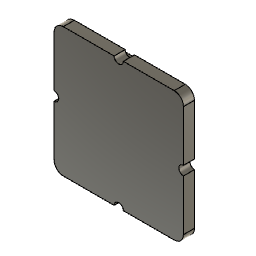
Coaster Holder with Coaster v3 (Autodesk Fusion 360 archive; units mm, degrees)
design "Coaster"
Autodesk Fusion 360 part; units mm, degrees
sketch "Sketch3" plane through (0, 0, 0) normal (0, 1, 0) x (1, 0, 0)
  line L0 (127, -127) -> (38.1, -127)
  line L1 (38.1, -127) -> (38.1, -38.1)
  line L2 (38.1, -38.1) -> (127, -38.1)
  line L3 (127, -38.1) -> (127, -127)
  line L4 (127, -82.55) -> (38.1, -82.55) construction
  dimension "d24" = 88.9
  dimension "d25" = 88.9
  constraint horizontal L0
  constraint vertical L1
  constraint horizontal L2
  constraint vertical L3
  constraint midpoint L3 L4.start
  constraint midpoint L1 L4.end
  measures "d24" distance of L0.start L0.end
  measures "d25" distance of L0.start L2.end
sketch "Sketch4" plane through (0, 0, 0) normal (0, 1, 0) x (1, 0, 0)
  line L0 (114.3445, -111.3227) -> (104.4288, -120.5494)
  line L1 (104.4288, -120.5494) -> (60.6138, -120.5494)
  line L2 (60.6138, -120.5494) -> (50.4318, -111.0618)
  line L3 (50.4318, -111.0618) -> (50.4318, -98.4259)
  line L4 (50.4318, -98.4259) -> (65.3763, -98.4259)
  line L5 (65.3763, -98.4259) -> (65.3763, -106.5936)
  line L6 (65.3763, -106.5936) -> (99.367, -106.5936)
  line L7 (99.367, -106.5936) -> (99.367, -90.3353)
  line L8 (99.367, -90.3353) -> (60.7032, -90.3353)
  line L9 (60.7032, -90.3353) -> (50.5442, -80.8012)
  line L10 (50.5442, -80.8012) -> (50.5442, -54.1925)
  line L11 (50.5442, -54.1925) -> (60.7032, -44.5506)
  line L12 (60.7032, -44.5506) -> (104.4543, -44.5506)
  line L13 (104.4543, -44.5506) -> (114.6143, -54.0756)
  line L14 (114.6143, -54.0756) -> (114.6143, -66.7756)
  line L15 (114.6143, -66.7756) -> (99.3743, -66.7756)
  line L16 (99.3743, -66.7756) -> (99.3108, -58.7746)
  line L17 (99.3108, -58.7746) -> (65.7193, -58.7746)
  line L18 (65.7193, -58.7746) -> (65.7193, -76.3006)
  line L19 (65.7193, -76.3006) -> (104.4543, -76.3006)
  line L20 (104.4543, -76.3006) -> (114.4555, -85.8256)
  line L21 (114.4555, -85.8256) -> (114.3445, -111.3227)
  line L22 (82.5213, -120.5494) -> (82.5787, -44.5506) construction
  line L23 (127, -82.55) -> (38.1, -82.55)
  constraint horizontal L12
  constraint midpoint L1 L22.start
  constraint midpoint L12 L22.end
  constraint midpoint L22 L23
extrude "Extrude5" add sketch "Sketch4" along normal blind 12.7 makes body 1
extrude "Extrude6" cut sketch "Sketch3" along normal blind 5.08 bodies 1
extrude "Extrude7" add sketch "Sketch4" sketch "Sketch3" along normal blind 7.62 of sketch 2 bodies 1
scale "Scale1" factor 1 about (127, 7.62, 127) bodies 1
sketch "Sketch7" plane through (0, 7.62, 0) normal (0, 1, 0) x (-1, 0, 0)
  line L0 (-127, 38.1) -> (-38.1, 38.1)
  line L1 (-38.1, 38.1) -> (-38.1, 127)
  line L2 (-38.1, 127) -> (-127, 127)
  line L3 (-127, 127) -> (-127, 38.1)
  line L4 (-50.5442, 80.8012) -> (-50.5442, 54.1925)
  line L5 (-50.5442, 54.1925) -> (-60.7032, 44.5506)
  line L6 (-60.7032, 44.5506) -> (-104.4543, 44.5506)
  line L7 (-104.4543, 44.5506) -> (-114.6143, 54.0756)
  line L8 (-114.6143, 54.0756) -> (-114.6143, 66.7756)
  line L9 (-114.6143, 66.7756) -> (-99.3743, 66.7756)
  line L10 (-99.3743, 66.7756) -> (-99.3108, 58.7746)
  line L11 (-99.3108, 58.7746) -> (-65.7193, 58.7746)
  line L12 (-65.7193, 58.7746) -> (-65.7193, 76.3006)
  line L13 (-65.7193, 76.3006) -> (-104.4543, 76.3006)
  line L14 (-104.4543, 76.3006) -> (-114.4555, 85.8256)
  line L15 (-114.4555, 85.8256) -> (-114.3445, 111.3227)
  line L16 (-114.3445, 111.3227) -> (-104.4288, 120.5494)
  line L17 (-104.4288, 120.5494) -> (-60.6138, 120.5494)
  line L18 (-60.6138, 120.5494) -> (-50.4318, 111.0618)
  line L19 (-50.4318, 111.0618) -> (-50.4318, 98.4259)
  line L20 (-50.4318, 98.4259) -> (-65.3763, 98.4259)
  line L21 (-65.3763, 98.4259) -> (-65.3763, 106.5936)
  line L22 (-65.3763, 106.5936) -> (-99.367, 106.5936)
  line L23 (-99.367, 106.5936) -> (-99.367, 90.3353)
  line L24 (-99.367, 90.3353) -> (-60.7032, 90.3353)
  line L25 (-60.7032, 90.3353) -> (-50.5442, 80.8012)
  line L26 (-127, 82.55) -> (-38.1, 82.55) construction
  line L27 (-82.55, 127) -> (-82.55, 38.1) construction
  circle A0 centre (-127, 82.55) radius 3.175
  circle A1 centre (-82.55, 127) radius 3.175
  circle A2 centre (-38.1, 82.55) radius 3.175
  circle A3 centre (-82.55, 38.1) radius 3.175
  dimension "d33" = 6.35
  dimension "d34" = 6.35
  dimension "d35" = 6.35
  dimension "d36" = 6.35
  constraint midpoint L3 L26.start
  constraint midpoint L1 L26.end
  constraint midpoint L2 L27.start
  constraint midpoint L0 L27.end
  constraint coincident L26.start A0.centre
  constraint coincident L27.start A1.centre
  constraint coincident L26.end A2.centre
  constraint coincident L27.end A3.centre
  measures "d33" diameter of A0
  measures "d34" diameter of A1
  measures "d35" diameter of A2
  measures "d36" diameter of A3
extrude "Extrude8" cut sketch "Sketch7" against normal blind 25.4 contours L0 A3 | L0 A3 | L1 A2 | L1 A2 | L3 A0 | L3 A0 | L2 A1 | L2 A1 bodies 1
fillet "Fillet2" radius 6.35 4 edges at (38.1, 3.81, 38.1) (38.1, 3.81, 127) (127, 3.81, 127) (127, 3.81, 38.1) on bodies 1
copy_body "Body->Comp1" bodies 1 removing the originals makes body 2 in component "Coaster"
sketch "Sketch8" plane through (0, 7.62, 0) normal (0, 1, 0) x (-1, 0, 0)
  arc A0 (-127, 44.45) -> (-120.65, 38.1) centre (-120.65, 44.45) ccw
  line L0 (-120.65, 38.1) -> (-85.725, 38.1)
  arc A1 (-79.375, 38.1) -> (-85.725, 38.1) centre (-82.55, 38.1) ccw
  line L1 (-79.375, 38.1) -> (-44.45, 38.1)
  arc A2 (-44.45, 38.1) -> (-38.1, 44.45) centre (-44.45, 44.45) ccw
  line L2 (-38.1, 44.45) -> (-38.1, 79.375)
  arc A3 (-38.1, 85.725) -> (-38.1, 79.375) centre (-38.1, 82.55) ccw
  line L3 (-38.1, 85.725) -> (-38.1, 120.65)
  arc A4 (-38.1, 120.65) -> (-44.45, 127) centre (-44.45, 120.65) ccw
  line L4 (-44.45, 127) -> (-79.375, 127)
  arc A5 (-85.725, 127) -> (-79.375, 127) centre (-82.55, 127) ccw
  line L5 (-85.725, 127) -> (-120.65, 127)
  arc A6 (-120.65, 127) -> (-127, 120.65) centre (-120.65, 120.65) ccw
  line L6 (-127, 120.65) -> (-127, 85.725)
  arc A7 (-127, 79.375) -> (-127, 85.725) centre (-127, 82.55) ccw
  line L7 (-127, 79.375) -> (-127, 44.45)
  line L8 (-50.5442, 80.8012) -> (-50.5442, 54.1925)
  line L9 (-50.5442, 54.1925) -> (-60.7032, 44.5506)
  line L10 (-60.7032, 44.5506) -> (-104.4543, 44.5506)
  line L11 (-104.4543, 44.5506) -> (-114.6143, 54.0756)
  line L12 (-114.6143, 54.0756) -> (-114.6143, 66.7756)
  line L13 (-114.6143, 66.7756) -> (-99.3743, 66.7756)
  line L14 (-99.3743, 66.7756) -> (-99.3108, 58.7746)
  line L15 (-99.3108, 58.7746) -> (-65.7193, 58.7746)
  line L16 (-65.7193, 58.7746) -> (-65.7193, 76.3006)
  line L17 (-65.7193, 76.3006) -> (-104.4543, 76.3006)
  line L18 (-104.4543, 76.3006) -> (-114.4555, 85.8256)
  line L19 (-114.4555, 85.8256) -> (-114.3445, 111.3227)
  line L20 (-114.3445, 111.3227) -> (-104.4288, 120.5494)
  line L21 (-104.4288, 120.5494) -> (-60.6138, 120.5494)
  line L22 (-60.6138, 120.5494) -> (-50.4318, 111.0618)
  line L23 (-50.4318, 111.0618) -> (-50.4318, 98.4259)
  line L24 (-50.4318, 98.4259) -> (-65.3763, 98.4259)
  line L25 (-65.3763, 98.4259) -> (-65.3763, 106.5936)
  line L26 (-65.3763, 106.5936) -> (-99.367, 106.5936)
  line L27 (-99.367, 106.5936) -> (-99.367, 90.3353)
  line L28 (-99.367, 90.3353) -> (-60.7032, 90.3353)
  line L29 (-60.7032, 90.3353) -> (-50.5442, 80.8012)
  line L30 (-82.55, 123.825) -> (-82.55, 41.275) construction
  line L31 (-88.9, 95.4942) -> (-76.2, 95.4942) construction
  line L32 (-76.2, 95.4942) -> (-76.2, 103.7702) construction
  line L33 (-76.2, 103.7702) -> (-88.9, 103.7702) construction
  line L34 (-88.9, 103.7702) -> (-88.9, 95.4942) construction
  line L35 (-86.364, 67.5718) -> (-78.7441, 67.5226) construction
  line L36 (-78.7441, 67.5226) -> (-78.6956, 75.0239) construction
  line L37 (-78.6956, 75.0239) -> (-86.3156, 75.0731) construction
  line L38 (-86.3156, 75.0731) -> (-86.364, 67.5718) construction
  text T0 "N" font "Arial" height 10 align centre top in box 12.7 x 8.276 at (-88.9, 95.4942) x (1, 0) y (0, 1) spacing 1 kerned
  text T1 "C" font "Arial" height 10 align centre top in box 7.6201 x 7.5014 at (-86.364, 67.5718) x (0.999979, -0.006455) y (0.006455, 0.999979) spacing 1 kerned
  constraint midpoint A5 L30.start
  constraint midpoint A1 L30.end
extrude "Extrude1" cut sketch "Sketch8" against normal blind 2.54 text T0 bodies 2 in component "Coaster"
extrude "Extrude2" cut sketch "Sketch8" against normal blind 2.54 text T1 bodies 2 in component "Coaster"
component "Coaster" placed x (1, 0, 0) y (0, 1, 0) z (0, 0, 1) at (0, 0, 0)
